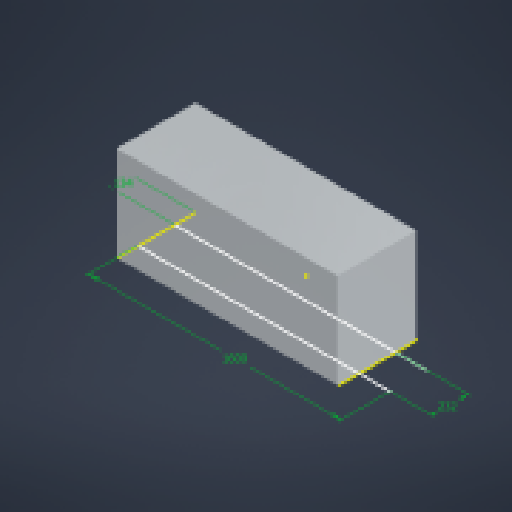
# Autodesk Inventor part: testhell
Saved by Autodesk Inventor 2023 (Build 270158000, 158)
## iProperties
Created: 2022-09-07
Part Number: testhell
Material: Steel, Mild
Document SubType Name: Modeling
Designer: Mike
Density: 7.85 g/cm^3
Appearance: Clear
Author: Mike
Autodesk Inventor part; units mm, degrees
ref_plane "YZ Plane" through (0, 0, 0) normal (1, 0, 0) x (0, 1, 0)
ref_plane "XZ Plane" through (0, 0, 0) normal (0, 1, 0) x (-1, 0, 0)
ref_plane "XY Plane" through (0, 0, 0) normal (0, 0, 1) x (1, 0, 0)
sketch "Sketch1" plane through (0, 0, 0) normal (0, 0, 1) x (1, 0, 0)
  line L0 (-700, 300) -> (700, 300)
  line L1 (700, 300) -> (700, -300)
  line L2 (700, -300) -> (-700, -300)
  line L3 (-700, -300) -> (-700, 300)
  line L4 (-700, 300) -> (700, -300) construction
  line L5 (700, 300) -> (-700, -300) construction
  point P0 (0, 0)
  dimension "d0" = 1400
  dimension "d1" = 600
  constraints: 12 end point, 2 midpoint, 2 parallel, 1 horizontal, 1 perpendicular
  measures "d0" distance of L1.end L2.end
  measures "d1" distance of L0.end L1.end
extrude "Extrusion1" add sketch "Sketch1" along normal blind 500
sketch "Sketch2" plane through (-700, -300, 0) normal (0, -1, 0) x (1, 0, 0)
  line L0 (0, 0) -> (0, 500) projected
  line L1 (0, 366) -> (1400, 366)
  line L2 (0, 134) -> (1400, 134)
  line L3 (1400, 0) -> (1400, 500) projected
  line L4 (1400, 134) -> (1600, 134)
  line L5 (1400, 366) -> (1600, 366)
  point P0 (700, 0)
  dimension "d4" = 134
  dimension "d5" = 232
  dimension "d6" = 1400
  dimension "d7" = 200
  constraints: 8 end point, 4 horizontal, 3 point on line
  measures "d4" distance from line of L2 L0.start
  measures "d5" distance between parallel lines of L1 L2
  measures "d6" distance of L1.start L1.end
  measures "d7" distance of L1.end L5.end
body "Solid1"
